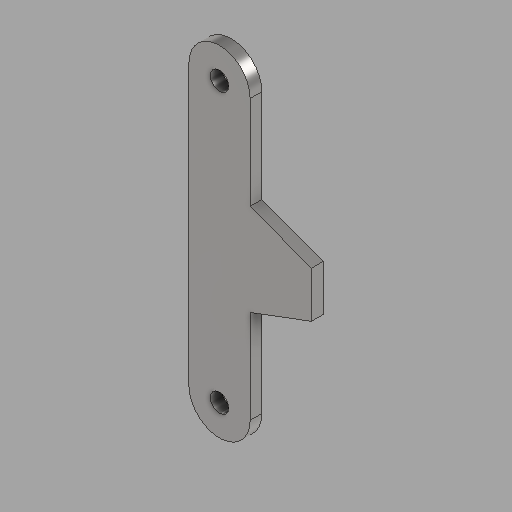
# Autodesk Inventor part: Eslabon de arrastre externo
Saved by Autodesk Inventor 2024.3 (Build 283343010, 343A)
## iProperties
Created: 2025-05-04
Part Number: Eslabon de arrastre externo
Material: Steel, Mild
Document SubType Name: Modeling
Designer: Gary
Density: 7.85 g/cm^3
Appearance: Semi-Polished
Author: Gary
Autodesk Inventor part; units mm, degrees
ref_plane "YZ Plane" through (0, 0, 0) normal (1, 0, 0) x (0, 1, 0)
ref_plane "XZ Plane" through (0, 0, 0) normal (0, 1, 0) x (-1, 0, 0)
ref_plane "XY Plane" through (0, 0, 0) normal (0, 0, 1) x (1, 0, 0)
sketch "Sketch1" plane through (0, 0, 0) normal (0, 0, 1) x (1, 0, 0)
  line L0 (0, 0) -> (0, 455) construction
  line L1 (50, 0) -> (50, 455)
  line L2 (-50, 455) -> (-50, 0)
  arc A0 (-50, 0) -> (50, 0) centre (0, 0) ccw
  arc A1 (50, 455) -> (-50, 455) centre (0, 455) ccw
  circle A2 centre (0, 455) radius 15
  circle A3 centre (0, 0) radius 15
  point P0 (0, 227.5)
  point P1 (0, 505)
  point P2 (0, -50)
  dimension "d0" = 455
  dimension "d2" = 30
  dimension "d3" = 30
  dimension "d6" = 555
  constraints: 8 end point, 6 point on circle, 4 centre point, 4 tangent, 2 coincident, 1 midpoint, 1 parallel, 1 vertical
  measures "d0" distance of L0.start L0.end
  measures "d2" diameter of A2
  measures "d3" diameter of A3
  measures "d6" distance of point (0, 505) point (0, -50)
extrude "Extrusion1" add sketch "Sketch1" along normal blind 12.7 and the other way blind 6.4
sketch "Sketch3" plane through (0, 0, 12.7) normal (0, 0, 1) x (1, 0, 0)
  line L0 (50, 0) -> (50, 455) projected
  line L1 (150, 227.5) -> (150, 265)
  line L2 (150, 265) -> (50, 302.5)
  line L3 (150, 227.5) -> (150, 190)
  line L4 (150, 190) -> (50, 152.5)
  point P0 (0, 0)
  point P1 (50, 227.5)
  dimension "d9" = 150
  dimension "d10" = 75
  dimension "d11" = 152.5
  dimension "d12" = 100
  constraints: 8 end point, 3 point on line, 2 equal length, 1 midpoint, 1 vertical
  measures "d9" distance of L2.end L4.end
  measures "d10" distance of L3.end L1.end
  measures "d11" vertical distance of point (0, 0) L4.end
  measures "d12" distance from line of L1 point (50, 227.5)
extrude "Extrusion2" add sketch "Sketch3" against normal blind 19.1
sketch "Sketch4" plane through (0, 0, -6.4) normal (0, 0, -1) x (-1, 0, 0)
  point P0 (0, 0)
body "Solid1"
